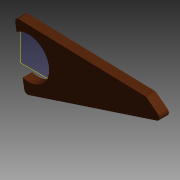
# Autodesk Inventor part: body07
Saved by Autodesk Inventor 2013 (Build 170138000, 138)
## iProperties
Created: 2013-02-19
Part Number: body07
Material: Wood (Walnut)
Document SubType Name: Modeling
Designer: Nano
Density: 0.55 g/cm^3
Mass: 9079.15 g
Surface Area: 6785.14 cm^2
Volume: 16507.6 cm^3
Author: Nano
Autodesk Inventor part; units mm, degrees
ref_plane "YZ Plane" through (0, 0, 0) normal (1, 0, 0) x (0, 1, 0)
ref_plane "XZ Plane" through (0, 0, 0) normal (0, 1, 0) x (-1, 0, 0)
ref_plane "XY Plane" through (0, 0, 0) normal (0, 0, 1) x (1, 0, 0)
ref_plane "Work Plane1" through (0, 0, -22.225) normal (0, 0, -1) x (-1, 0, 0)
sketch "Sketch1" plane through (0, 0, -22.225) normal (0, 0, -1) x (-1, 0, 0)
  arc A0 (88.9626, 123.799) -> (43.8693, -146.1511) centre (0.2092, -0.1167) ccw
  line L0 (104.0584, 214.2592) -> (-870.0682, 186.8193)
  line L1 (-870.0682, 186.8193) -> (-996.5964, 89.8924)
  line L2 (-996.5964, 89.8924) -> (27.3448, -245.173)
  line L3 (104.0584, 214.2592) -> (88.9626, 123.799)
  line L4 (27.3448, -245.173) -> (43.8693, -146.1511)
  constraints: 11 end point, 2 point on circle, 1 centre point
extrude "Extrusion1" add sketch "Sketch1" against normal blind 69.85
fillet "Fillet1" radius 25.4 1 edges at (-104.0584, 214.2592, 12.7)
fillet "Fillet2" radius 25.4 1 edges at (-27.3448, -245.173, 12.7)
fillet "Fillet3" radius 25.4 2 edges at (996.5964, 89.8924, 12.7) (870.0682, 186.8193, 12.7)
body "Solid1"
